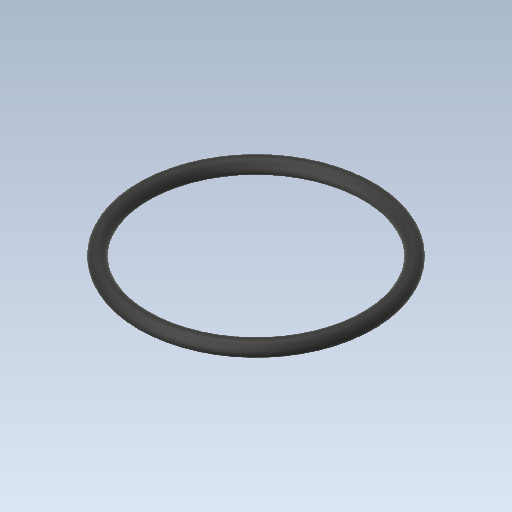
# Autodesk Inventor part: #22 O-ring
Saved by Autodesk Inventor 2020 (Build 240168000, 168)
## iProperties
Created: 2017-11-13
Part Number: #22 O-ring
Material: Thermoplastic Resin
Document SubType Name: Modeling
Designer: Alex
Mass: 0.268561 g
Surface Area: 4.72021 cm^2
Volume: 0.209813 cm^3
Density: 1.28 g/cm^3
Appearance: Smooth - Black
Catalog Web Link: https://www.amazon.com/gp/product/B000FMYRGG/ref=oh_aui_search_detailpage?ie=UTF8&psc=1
Description: #22 Silicone O-ring
Vendor: Amazon
Author: Alex
Autodesk Inventor part; units mm, degrees
ref_plane "YZ Plane" through (0, 0, 0) normal (1, 0, 0) x (0, 1, 0)
ref_plane "XZ Plane" through (0, 0, 0) normal (0, 1, 0) x (-1, 0, 0)
ref_plane "XY Plane" through (0, 0, 0) normal (0, 0, 1) x (1, 0, 0)
sketch "Sketch1" plane through (0, 0, 0) normal (0, 0, 1) x (1, 0, 0)
  circle A0 centre (13.4493, 0) radius 0.889
  line L0 (0, -1.2446) -> (0, 1.2446) projected
  point P0 (0, 0)
  dimension "d0" = 1.778
  dimension "d1" = 13.4493
  constraints: 1 centre point, 1 horizontal alignment
  measures "d0" diameter of A0
  measures "d1" distance of A0.centre point (0, 0)
revolve "Revolution1" add sketch "Sketch1" angle 360 about axis through (0, -10, 0) along (0, 1, 0)
body "Solid1"
